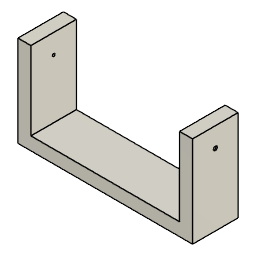
Solar Platform (Autodesk Fusion 360 design; units mm, degrees)
Autodesk Fusion 360 part; units mm, degrees
sketch "Sketch1" plane through (0, 0, 0) normal (0, 1, 0) x (1, 0, 0)
  line L0 (-67, -114.8999) -> (-57, -114.8999)
  line L1 (-57, -114.8999) -> (-57, -54.8999)
  line L2 (-57, -54.8999) -> (57, -54.8999)
  line L3 (57, -54.8999) -> (57, -114.8999)
  line L4 (57, -114.8999) -> (67, -114.8999)
  line L5 (67, -114.8999) -> (67, -44.8999)
  line L6 (67, -44.8999) -> (-67, -44.8999)
  line L7 (-67, -44.8999) -> (-67, -114.8999)
  dimension "d2" = 67
  dimension "d3" = 10
  dimension "d6" = 70
  dimension "d16" = 10
  dimension "d17" = 10
  dimension "d31" = 67
  constraint horizontal L0
  constraint perpendicular L0 L1
  constraint perpendicular L1 L2
  constraint perpendicular L2 L3
  constraint perpendicular L3 L4
  constraint perpendicular L2 L5
  constraint perpendicular L5 L6
  constraint perpendicular L0 L7
  constraint equal L0 L4
  constraint equal L5 L7
  measures "d2" distance of origin L7
  measures "d3" distance of L2 L6
  measures "d6" distance of L0.start L6.end
  measures "d16" distance of L0.start L0.end
  measures "d17" distance of L3.end L4.end
  measures "d31" horizontal distance of origin L5.end
extrude "Extrude1" add sketch "Sketch1" along normal blind 35
sketch "Sketch3" plane through (-67, 0, 0) normal (-1, 0, 0) x (0, -1, 0)
  line L0 (0, 44.8999) -> (0, 114.8999)
  line L1 (0, 114.8999) -> (-35, 114.8999)
  line L2 (-35, 114.8999) -> (-35, 44.8999)
  line L3 (-35, 44.8999) -> (0, 44.8999)
  circle A0 centre (-17.5, 99.8999) radius 1
  dimension "d12" = 2
  dimension "d15" = 17.5
  dimension "d24" = 15
  measures "d12" diameter of A0
  measures "d15" distance of L0 A0.centre
  measures "d24" distance of L1 A0.centre
extrude "Extrude2" cut sketch "Sketch3" against normal blind 101 contours A0
sketch "Sketch4" plane through (0, 35, 0) normal (0, 1, 0) x (-1, 0, 0)
  line L0 (67, 44.8999) -> (67, 114.8999)
  line L1 (67, 114.8999) -> (57, 114.8999)
  line L2 (57, 114.8999) -> (57, 54.8999)
  line L3 (57, 54.8999) -> (-57, 54.8999)
  line L4 (-57, 54.8999) -> (-57, 114.8999)
  line L5 (-57, 114.8999) -> (-67, 114.8999)
  line L6 (-67, 114.8999) -> (-67, 44.8999)
  line L7 (-67, 44.8999) -> (67, 44.8999)
  line L8 (-5, 52.3999) -> (1, 52.3999)
  line L9 (1, 52.3999) -> (1, 47.3999)
  line L10 (1, 47.3999) -> (-5, 47.3999)
  line L11 (-5, 47.3999) -> (-5, 52.3999)
  line L12 (-5, 52.3999) -> (1, 47.3999) construction
  line L13 (1, 52.3999) -> (-5, 47.3999) construction
  point P0 (-2, 49.8999)
  dimension "d18" = 5
  dimension "d19" = 6
  dimension "d20" = 5
  dimension "d21" = 65
  constraint horizontal L8
  constraint perpendicular L8 L9
  constraint parallel L8 L10
  constraint parallel L9 L11
  constraint coincident L12 P0
  constraint coincident L13 P0
  measures "d18" distance of L8.end L9.end
  measures "d19" distance of L9.end L10.end
  measures "d20" distance of L7 P0
  measures "d21" distance of L6 P0
extrude "Extrude3" cut sketch "Sketch4" against normal blind 20 contours L8 L9 L10 L11
mirror "Mirror2" about plane through (0, 0, 0) normal (1, 0, 0) of "Extrude2"
fillet "Fillet2" radius 0.5 2 edges at (67, 18.4323, 99.5383) (-67, 18.4323, 100.2615)
